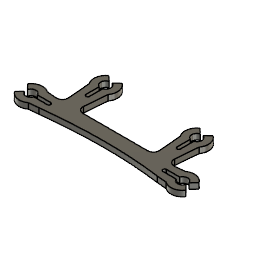
Piesa_5_suport (Autodesk Fusion 360 design; units mm, degrees)
part number: 2026-05-31-14-37-00-201
part number: 2026-05-31-16-38-22-754
Autodesk Fusion 360 part; units mm, degrees
note: some values were not read from the file. Set by a fixed rule: which sketch regions a step uses.
sketch "top view" plane through (0, 0, 0) normal (0, 0, 1) x (1, 0, 0)
  line L0 (-105, 33) -> (-105, -11) construction
  line L1 (-125, 15) -> (-126.282, 15) construction
  line L2 (-126.282, 15) -> (-126.282, 15.368) construction
  line L3 (-126.282, 15.368) -> (-127.5617, 16.726)
  line L4 (-126.282, 15.368) -> (-124.416, 15.368) construction
  line L5 (-127.5617, 16.726) -> (-127.5786, 16.744)
  line L6 (-126.282, 14.632) -> (-127.5617, 13.274)
  line L7 (-127.5617, 13.274) -> (-127.5786, 13.256)
  line L8 (-125, 15) -> (-123.748, 15) construction
  line L9 (-123.748, 15) -> (-123.748, 17.8501) construction
  line L10 (-123.748, 15) -> (-123.748, 12.1499) construction
  line L11 (-123.748, 15) -> (-123.748, 15.461) construction
  line L12 (-123.748, 15) -> (-123.748, 14.539) construction
  arc A0 (-126.282, 14.632) -> (-123.7484, 14.539) centre (-125, 15) ccw
  arc A1 (-123.7484, 15.461) -> (-126.282, 15.368) centre (-125, 15) ccw
  line L13 (-121.9213, 15.461) -> (-120.224, 15.461)
  line L14 (-121.9213, 14.539) -> (-120.224, 14.539)
  arc A2 (-127.5786, 13.256) -> (-123.134, 12.5083) centre (-125, 15) ccw
  arc A3 (-123.134, 17.4917) -> (-127.5786, 16.744) centre (-125, 15) ccw
  arc A4 (-120.224, 14.539) -> (-120.224, 15.461) centre (-120.224, 15) ccw
  line L15 (-125, 15) -> (-123.134, 15) construction
  line L16 (-123.134, 15) -> (-123.134, 17.4917) construction
  line L17 (-123.134, 17.4917) -> (-120.5917, 17.2693)
  line L18 (-123.134, 17.4917) -> (-120.582, 17.4917) construction
  line L19 (-123.134, 12.5083) -> (-120.5917, 12.7307)
  line L20 (-118.9667, 18.8943) -> (-119.4889, 24.8635)
  line L21 (-118.9667, 18.8943) -> (-111.0132, 18.8943) construction
  line L22 (-123.134, 17.4917) -> (-118.737, 17.4917) construction
  line L23 (-118.9667, 18.8942) -> (-118.9667, 18.8942)
  arc A5 (-120.5917, 17.2693) -> (-118.9667, 18.8943) centre (-120.461, 18.7636) ccw
  line L24 (-119.4004, 17.7029) -> (-121.3897, 15.7137) construction
  line L25 (-119.4004, 17.7029) -> (-116.4958, 14.7981) construction
  line L26 (-123.748, 15.461) -> (-121.9213, 15.461)
  line L27 (-123.748, 14.539) -> (-121.9213, 14.539)
  arc A6 (-117.4582, 21.9535) -> (-116.9972, 21.4925) centre (-116.9972, 21.9535) ccw
  line L28 (-116.9972, 20.106) -> (-116.9972, 11.6268) construction
  arc A7 (-115.0277, 18.8943) -> (-113.4026, 17.2693) centre (-113.5334, 18.7636) ccw
  line L29 (-113.4026, 17.2693) -> (-105, 17.2693)
  line L30 (-105, 33) -> (-105, -11) construction
  line L31 (-96.5974, 17.2693) -> (-105, 17.2693)
  arc A8 (-96.5974, 17.2693) -> (-94.9723, 18.8943) centre (-96.4667, 18.7636) ccw
  line L32 (-94.9723, 18.8943) -> (-95.2773, 22.3803)
  line L33 (-93.0028, 20.106) -> (-93.0028, 11.6268) construction
  line L34 (-91.7911, 18.8943) -> (-98.9868, 18.8943) construction
  line L35 (-91.0333, 17.2692) -> (-93.5042, 14.7981) construction
  line L36 (-91.0333, 17.4917) -> (-91.263, 17.4917) construction
  line L37 (-82.4383, 16.726) -> (-82.4214, 16.744)
  line L38 (-83.718, 15) -> (-83.718, 15.368) construction
  arc A9 (-86.866, 12.5083) -> (-86.252, 12.1499) centre (-85, 15) ccw
  line L39 (-91.0333, 18.8943) -> (-91.0333, 18.8943)
  line L40 (-82.4383, 13.274) -> (-82.4214, 13.256)
  spline S0 degree 5 poles (-120.5917, 12.7307) (-119.326, 12.8736) (-116.8026, 13.1337) (-113.042, 13.4467) (-108.0773, 13.7071) (-101.9596, 13.7532) (-97.0107, 13.5402) (-93.3168, 13.2188) (-90.8349, 12.9243) (-89.5363, 12.7482) (-89.4083, 12.7307) knots 0 0 0 0 0 0 0.1 0.2 0.3 0.4 0.5 0.51094 0.51094 0.51094 0.51094 0.51094 0.51094
  line L41 (-92.4447, 13.1474) -> (-86.3719, 12.3139)
  line L42 (-123.748, 14.539) -> (-123.7484, 14.539)
  line L43 (-123.748, 15.461) -> (-123.7484, 15.461)
  line L44 (-116.5362, 25.4775) -> (-116.5362, 25.4779)
  line L45 (-117.4582, 25.4775) -> (-117.4582, 25.4779)
  line L46 (-115.0277, 18.8943) -> (-115.0278, 18.8929)
  line L47 (-118.9704, 18.9365) -> (-118.9667, 18.8943)
  line L48 (-119.4004, 17.7029) -> (-116.9972, 20.106) construction
  line L49 (-125, 15) -> (-93.0028, 15) construction
  line L50 (-93.0028, 15) -> (-125, 15) construction
  line L51 (-91.7911, 18.8943) -> (-93.0028, 20.106) construction
  arc A10 (-114.5054, 24.8635) -> (-115.2532, 29.3081) centre (-116.9972, 26.7295) ccw
  arc A11 (-118.7411, 29.3081) -> (-119.4889, 24.8635) centre (-116.9972, 26.7295) ccw
  arc A12 (-117.3652, 28.0115) -> (-117.4582, 25.4779) centre (-116.9972, 26.7295) ccw
  arc A13 (-116.5362, 25.4779) -> (-116.6292, 28.0115) centre (-116.9972, 26.7295) ccw
  line L52 (-116.5362, 23.6508) -> (-116.5362, 21.9535)
  arc A14 (-117.4582, 21.9535) -> (-116.5362, 21.9535) centre (-116.9972, 21.9535) ccw
  line L53 (-117.4582, 23.6508) -> (-117.4582, 21.9535)
  line L54 (-116.5362, 25.4779) -> (-116.5362, 23.6508)
  line L55 (-117.4582, 25.4779) -> (-117.4582, 23.6508)
  line L56 (-115.2532, 29.3081) -> (-116.6292, 28.0115)
  line L57 (-117.3652, 28.0115) -> (-118.7411, 29.3081)
  line L58 (-114.5054, 24.8635) -> (-115.0278, 18.8929)
  arc A15 (-90.5111, 24.8635) -> (-91.2589, 29.3081) centre (-93.0028, 26.7295) ccw
  arc A16 (-94.7468, 29.3081) -> (-95.4946, 24.8635) centre (-93.0028, 26.7295) ccw
  line L59 (-94.7468, 29.3081) -> (-93.3708, 28.0115)
  line L60 (-92.6348, 28.0115) -> (-91.2589, 29.3081)
  arc A17 (-92.5418, 25.4779) -> (-92.6348, 28.0115) centre (-93.0028, 26.7295) ccw
  arc A18 (-93.3708, 28.0115) -> (-93.4638, 25.4779) centre (-93.0028, 26.7295) ccw
  line L61 (-93.4638, 25.4779) -> (-93.4638, 23.6508)
  line L62 (-92.5418, 25.4779) -> (-92.5418, 23.6508)
  line L63 (-91.0333, 18.8943) -> (-90.5111, 24.8635)
  line L64 (-92.5418, 23.6508) -> (-92.5418, 21.9535)
  line L65 (-93.4638, 23.6508) -> (-93.4638, 21.9535)
  arc A19 (-93.4638, 21.9535) -> (-92.5418, 21.9535) centre (-93.0028, 21.9535) ccw
  arc A20 (-91.0333, 18.8943) -> (-89.4083, 17.2693) centre (-89.539, 18.7636) ccw
  line L66 (-86.866, 17.4917) -> (-89.4083, 17.2693)
  arc A21 (-82.4214, 16.744) -> (-86.866, 17.4917) centre (-85, 15) ccw
  arc A22 (-83.718, 15.368) -> (-86.2516, 15.461) centre (-85, 15) ccw
  arc A23 (-86.2516, 14.539) -> (-83.718, 14.632) centre (-85, 15) ccw
  arc A24 (-86.866, 12.5083) -> (-82.4214, 13.256) centre (-85, 15) ccw
  line L67 (-88.0787, 14.539) -> (-89.776, 14.539)
  line L68 (-88.0787, 15.461) -> (-89.776, 15.461)
  arc A25 (-89.776, 15.461) -> (-89.776, 14.539) centre (-89.776, 15) ccw
  line L69 (-95.4946, 24.8635) -> (-94.9722, 18.8929)
  line L70 (-86.866, 12.5083) -> (-89.4083, 12.7307)
  line L71 (-88.0787, 15.461) -> (-86.2516, 15.461)
  line L72 (-88.0787, 14.539) -> (-86.2516, 14.539)
  line L73 (-83.718, 15.368) -> (-82.4214, 16.744)
  line L74 (-83.718, 14.632) -> (-82.4214, 13.256)
  point P0 (-95.4946, 24.8635)
  point P1 (-94.7468, 29.3081)
  point P2 (-93.0028, 26.7295)
  point P3 (-88.6103, 15.7137)
  dimension "d3" = 6.226
  dimension "d4" = 1.282
  dimension "d5" = 0.368
  dimension "d6" = 133.3
  dimension "d7" = 1.866
  dimension "d8" = 1.252
  dimension "d9" = 0.461
  dimension "d10" = 0.461
  dimension "d11" = 3.524
  dimension "d12" = 0.922
  dimension "d13" = 1.866
  dimension "d14" = 2.552
  dimension "d15" = 5
  dimension "d16" = 3
  dimension "d17" = 95
  dimension "d18" = 5.992
  dimension "d20" = 4.397
  dimension "d24" = 0.922
  dimension "d25" = 6.226
  dimension "d28" = 0.922
  constraint horizontal L49
  constraint coincident L1.start L8.start
  constraint perpendicular L0 L49
  constraint concentric A0 A2
  constraint perpendicular L0 L1
  constraint perpendicular L1 L2
  constraint horizontal L4
  constraint parallel L3 L5
  constraint symmetric L1 L2.end L6.start
  constraint symmetric L1 L3.end L6.end
  constraint parallel L6 L7
  constraint parallel L8 L49
  constraint coincident L9.end A3
  constraint perpendicular L9 L49
  constraint coincident L10.end A2
  constraint perpendicular L10 L49
  constraint perpendicular L11 L49
  constraint perpendicular L8 L12
  constraint concentric A0 A1
  constraint perpendicular L9 L13
  constraint symmetric L13.end L14.end L49
  constraint coincident A4.centre L49
  constraint concentric A2 A3
  constraint parallel L15 L49
  constraint perpendicular L16 L49
  constraint horizontal L18
  constraint symmetric A3.start A2.end L49
  constraint symmetric L17.end L19.end L49
  constraint tangent L17 A5
  constraint horizontal L21
  constraint horizontal L22
  constraint coincident L20.start L21.start
  constraint coincident L20.start A5
  constraint midpoint A5 L24.start
  constraint tangent A5 L48
  constraint tangent A5 L24
  constraint perpendicular L24 L25
  constraint perpendicular L12 L27
  constraint perpendicular L28 L49
  constraint symmetric L17.end L28 A7.end
  constraint symmetric L20.start L28 A7.start
  constraint symmetric A5 L28 A7
  constraint coincident L0 L29.end
  constraint perpendicular L0 L29
  constraint symmetric L30.start L0 L0.start
  constraint symmetric L30.end L0 L0.end
  constraint symmetric L0 L1.end L38.start
  constraint symmetric L0 L2.end L38.end
  constraint symmetric L0 L3.end L37.start
  constraint symmetric L0 L5.end L37.end
  constraint symmetric L0 L6.end L40.start
  constraint symmetric L0 L7.end L40.end
  constraint symmetric L0 L10.end A9.end
  constraint symmetric L0 A2 A9
  constraint symmetric L0 A2.end A9.start
  constraint symmetric L0 L19.end S0.end
  constraint symmetric L0 L21.end L34.end
  constraint symmetric L0 L20.start L39.start
  constraint symmetric L0 L22.end L36.end
  constraint symmetric L0 L25.end L35.end
  constraint symmetric L0 L28.end L33.end
  constraint symmetric L0 A7.end L31.start
  constraint symmetric L0 A7.start A8.end
  constraint symmetric L0 A7 A8
  constraint symmetric L0 L29.end L31.end
  constraint midpoint S0.end L41
  constraint perpendicular L12 L42
  constraint parallel L26 L43
  constraint coincident A7 L46.end
  constraint coincident L20 L47.start
  constraint parallel L20 L47
  constraint coincident L33 L49.end
  constraint concentric A11 A12
  constraint concentric A12 A13
  constraint concentric A10 A11
  constraint parallel L52 L54
  constraint parallel L53 L55
  constraint tangent A14 L53
  constraint tangent L52 A14
  constraint symmetric L0 L6.start A23.end
  constraint symmetric L0 A0 A23
  constraint symmetric L0 A1 A22
  constraint symmetric L0 L13.end L68.end
  constraint symmetric L0 L14.end L67.end
  constraint symmetric L0 L13.start L68.start
  constraint symmetric L0 A2 A24
  constraint symmetric L0 A3 A21
  constraint symmetric L0 L14.start L67.start
  constraint symmetric L0 A4 A25
  constraint symmetric L0 A3.start L66.start
  constraint symmetric L0 L17.end A20.end
  constraint symmetric L0 L20.end A15.start
  constraint symmetric L0 A5 A20
  constraint symmetric L0 L24.end P3
  constraint symmetric L0 A0.end A23.start
  constraint symmetric L0 A1.start A22.end
  constraint symmetric L0 L45.end A17.start
  constraint symmetric L0 L44.end A18.end
  constraint symmetric L0 A13.end L59.end
  constraint symmetric L0 A10.end P1
  constraint symmetric L0 A12.start L60.start
  constraint symmetric L0 A11.start A15.end
  constraint symmetric L0 L52.end L65.end
  constraint symmetric L0 L52.start L61.end
  constraint symmetric L0 L53.start L62.end
  constraint symmetric L0 A6.start L64.end
  constraint symmetric L0 A10.start P0
  constraint symmetric L0 A10 A16
  constraint symmetric L0 A11 A15
  constraint symmetric L0 A12 A17
  constraint symmetric L0 A13 A18
  constraint symmetric L0 A14 A19
  constraint symmetric A2.end L30 A9.start
  constraint symmetric L19.end L30 S0.end
  constraint symmetric L30 L46.end L69.end
  constraint symmetric L30 A10.start P0
  constraint parallel L68 L71
  measures "d3" diameter of A2
  measures "d4" distance of L1.start L1.end
  measures "d5" distance of L1.end L2.end
  measures "d6" angle of L3 L4
  measures "d7" distance of L2.end L3.end
  measures "d8" distance of L1.start L8.end
  measures "d9" distance of L8.end L11.end
  measures "d10" distance of L8.end L12.end
  measures "d11" distance of L11.end L13.end
  measures "d12" diameter of A4
  measures "d13" distance of L1.start L15.end
  measures "d14" distance of A3.start L17.end
  measures "d15" angle of L17 L18
  measures "d16" diameter of A5
  measures "d17" angle of L20 L21
  measures "d18" distance of L20.start L20.end
  measures "d20" distance of A3.start L20.start
  measures "d24" diameter of A6
  measures "d25" diameter of A11
  measures "d28" diameter of A14
extrude "Extrude1" add sketch "top view" along normal blind 1.5 contours L3 L5 L6 L7 A0 A1 L13 L14 A2 A3 A4 L17 L19 L20 A5 L26 L27 A6 A7 L29 L31 A8 L32 L37 A9 L40 S0 L47 A10 A11 A12 A13 L52 A14 L53 L54 L55 L56 L57 L58 A15 A16 L59 L60 A17 A18 L61 L62 L63 L64 L65 A19 A20 L66 A21 A22 A23 A24 L67 L68 A25 L69 L70 L71 L72 L73 L74 makes body 1
copy_body "Body->Comp1" bodies 1 removing the originals makes body 2 in component "Piesa_5 (1)"
component "Piesa_5 (1)" placed x (1, 0, 0) y (0, 1, 0) z (0, 0, 1) at (0, 0, 0)
equation "d3 = 3.113 mm + 3.113 mm"
equation "d12 = 0.461 mm + 0.461 mm"
equation "d24 = 0.461 mm + 0.461 mm"
equation "d25 = 3.113 mm + 3.113 mm"
equation "d28 = 0.461 mm + 0.461 mm"
named bodies: "corp piesa 5"
